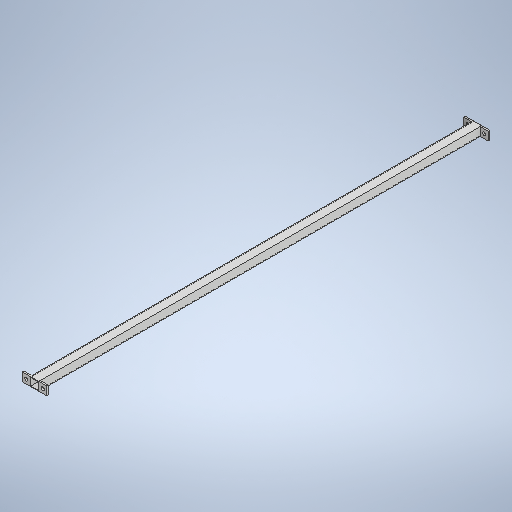
# Autodesk Inventor part: Bases_Perfiles_Acero
Saved by Autodesk Inventor 2025.2 (Build 292293000, 293)
## iProperties
Created: 2025-05-31
Part Number: Bases_Perfiles_Acero
Material: Generic
Document SubType Name: Modeling
Designer: USER
Density: 1 g/cm^3
Appearance: Default
Author: USER
Autodesk Inventor part; units mm, degrees
ref_plane "YZ Plane" through (0, 0, 0) normal (1, 0, 0) x (0, 1, 0)
ref_plane "XZ Plane" through (0, 0, 0) normal (0, 1, 0) x (-1, 0, 0)
ref_plane "XY Plane" through (0, 0, 0) normal (0, 0, 1) x (1, 0, 0)
sketch "Sketch2" plane through (0, 0, 0) normal (0, 0, 1) x (1, 0, 0)
  line L0 (0, 0) -> (31.75, 0)
  line L1 (31.75, 0) -> (31.75, 31.75)
  line L2 (31.75, 31.75) -> (0, 31.75)
  line L3 (0, 31.75) -> (0, 0)
  line L4 (2, 29.75) -> (29.75, 29.75)
  line L5 (29.75, 29.75) -> (29.75, 2)
  line L6 (29.75, 2) -> (2, 2)
  line L7 (2, 2) -> (2, 29.75)
  dimension "d0" = 31.75
  dimension "d1" = 31.75
  dimension "d2" = 2
  constraints: 16 end point, 4 parallel, 2 perpendicular, 1 horizontal, 3 other
  measures "d0" distance of L2.end L1.end
  measures "d1" distance of L1.end L0.end
  measures "d2" distance between parallel lines of L2 L4
extrude "Extrusion1" add sketch "Sketch2" along normal blind 1650
sketch "Sketch3" plane through (0, 0, 1650) normal (0, 0, 1) x (1, 0, 0)
  line L0 (31.75, 31.75) -> (0, 31.75) projected
  line L1 (0, 31.75) -> (-30, 31.75)
  line L2 (-30, 31.75) -> (-30, 0)
  line L3 (-30, 0) -> (0, 0)
  line L4 (0, 0) -> (0, 31.75)
  line L5 (31.75, 31.75) -> (61.75, 31.75)
  line L6 (61.75, 31.75) -> (61.75, 0)
  line L7 (61.75, 0) -> (31.75, 0)
  line L8 (31.75, 0) -> (31.75, 31.75)
  circle A0 centre (-15, 15.875) radius 6
  circle A1 centre (46.75, 15.875) radius 6
  dimension "d5" = 30
  dimension "d6" = 30
  dimension "d7" = 12
  dimension "d8" = 12
  constraints: 16 end point, 4 parallel, 2 centre point, 2 horizontal, 2 perpendicular, 1 point on line
  measures "d5" distance of L3.end L2.end
  measures "d6" distance of L6.end L7.end
  measures "d7" diameter of A0
  measures "d8" diameter of A1
extrude "Extrusion2" add sketch "Sketch3" against normal blind 6
sketch "Sketch4" plane through (0, 0, 0) normal (0, 0, -1) x (-1, 0, 0)
  line L0 (-61.75, 31.75) -> (30, 31.75) projected
  line L1 (30, 0) -> (-61.75, 0) projected
  line L2 (0, 31.75) -> (30, 31.75)
  line L3 (30, 31.75) -> (30, 0)
  line L4 (30, 0) -> (0, 0)
  line L5 (0, 0) -> (0, 31.75)
  line L6 (-31.75, 31.75) -> (-31.75, 0) projected
  line L7 (-31.75, 31.75) -> (-61.75, 31.75)
  line L8 (-61.75, 31.75) -> (-61.75, 0)
  line L9 (-61.75, 0) -> (-31.75, 0)
  line L10 (-31.75, 0) -> (-31.75, 31.75)
  circle A0 centre (-46.75, 15.875) radius 6 projected
  circle A1 centre (-46.75, 15.875) radius 6
  circle A2 centre (15, 15.875) radius 6
  dimension "d11" = 30
  dimension "d12" = 12
  constraints: 16 end point, 4 parallel, 2 centre point, 2 horizontal, 2 perpendicular, 2 point on line, 1 coincident
  measures "d11" distance of L9.end L8.end
  measures "d12" diameter of A1
extrude "Extrusion3" add sketch "Sketch4" against normal blind 6 contours L0 L6 L1 L8 | L0 L3 L1 L5
body "Solid1"
